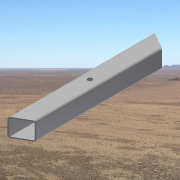
# Autodesk Inventor part: 2f2ao
Saved by Autodesk Inventor 2013 SP2 (Build 170200200, 200)
## iProperties
Company: HERA Project
Created: 2013-06-27
Part Number: 2f2ao
Material: Steel
Document SubType Name: Modeling
Designer: David DeBoer
Density: 7.85 g/cm^3
Mass: 221.444 g
Surface Area: 345.852 cm^2
Volume: 28.2094 cm^3
Description: Feed backplane support cross piece
Title: Backplane support piece
Author: David DeBoer
Autodesk Inventor part; units mm, degrees
ref_plane "YZ Plane" through (0, 0, 0) normal (1, 0, 0) x (0, 1, 0)
ref_plane "XZ Plane" through (0, 0, 0) normal (0, 1, 0) x (-1, 0, 0)
ref_plane "XY Plane" through (0, 0, 0) normal (0, 0, 1) x (1, 0, 0)
sketch "Sketch1" plane through (0, 0, 0) normal (0, 0, 1) x (1, 0, 0)
  line L0 (3.175, 0) -> (22.225, 0)
  line L1 (25.4, 3.175) -> (25.4, 22.225)
  line L2 (22.225, 25.4) -> (3.175, 25.4)
  line L3 (0, 22.225) -> (0, 3.175)
  arc A0 (3.175, 25.4) -> (0, 22.225) centre (3.175, 22.225) ccw
  arc A1 (0, 3.175) -> (3.175, 0) centre (3.175, 3.175) ccw
  arc A2 (22.225, 0) -> (25.4, 3.175) centre (22.225, 3.175) ccw
  arc A3 (25.4, 22.225) -> (22.225, 25.4) centre (22.225, 22.225) ccw
  line L4 (3.175, 23.749) -> (22.225, 23.749)
  arc A4 (23.749, 22.225) -> (22.225, 23.749) centre (22.225, 22.225) ccw
  line L5 (23.749, 22.225) -> (23.749, 3.175)
  arc A5 (22.225, 1.651) -> (23.749, 3.175) centre (22.225, 3.175) ccw
  line L6 (22.225, 1.651) -> (3.175, 1.651)
  arc A6 (1.651, 3.175) -> (3.175, 1.651) centre (3.175, 3.175) ccw
  line L7 (1.651, 3.175) -> (1.651, 22.225)
  arc A7 (3.175, 23.749) -> (1.651, 22.225) centre (3.175, 22.225) ccw
  point P0 (0, 0)
  point P1 (25.4, 0)
  point P2 (0, 25.4)
  dimension "d0" = 25.4
  dimension "d1" = 25.4
  dimension "d2" = 3.175
  dimension "d3" = 1.651
  constraints: 16 end point, 16 point on circle, 8 centre point, 8 tangent, 6 point on line, 4 parallel, 3 equal radius, 2 perpendicular, 1 horizontal, 7 other
  measures "d0" distance of point (0, 0) point (25.4, 0)
  measures "d1" distance of point (0, 25.4) point (0, 0)
  measures "d2" radius of A0
  measures "d3" distance between parallel lines of L4 L2
extrude "Extrusion1" add sketch "Sketch1" along normal blind 203.2
sketch "Sketch2" plane through (3.175, 25.4, 0) normal (0, 1, 0) x (1, 0, 0)
  line L0 (19.05, -203.2) -> (0, -203.2) projected
  line L1 (-3.175, 0) -> (22.2557, 0)
  line L2 (-3.175, 0) -> (32.385, 0) construction
  line L3 (22.2557, 0) -> (22.2557, -14.6824)
  line L4 (-3.175, 0) -> (22.2557, -14.6824)
  line L5 (-3.175, 0) -> (-3.175, -203.2) construction
  line L6 (-3.175, -101.6) -> (22.2557, -101.6) construction
  line L7 (-3.175, -203.2) -> (22.2557, -203.2)
  line L8 (22.2557, -203.2) -> (22.2557, -188.5176)
  line L9 (-3.175, -203.2) -> (22.2557, -188.5176)
  point P0 (0, 0)
  constraints: 18 end point, 2 parallel, 2 perpendicular, 2 symmetric about line, 1 horizontal, 1 midpoint
extrude "Extrusion2" cut sketch "Sketch2" against normal blind 203.2
sketch "Sketch3" plane through (3.175, 25.4, 201.3669) normal (0, 1, 0) x (1, 0, 0)
  line L0 (0, 199.5338) -> (0, 0) projected
  line L1 (19.05, 188.5353) -> (19.05, 10.9985) projected
  line L2 (0, 99.7669) -> (19.05, 99.7669) construction
  circle A0 centre (9.525, 99.7669) radius 2.5512
  point P0 (-3.175, 201.3669)
  constraints: 3 midpoint, 2 end point, 1 centre point
hole "Hole1" at (12.7, 25.4, 101.6) direction (0, -1, 0) diameter 6.35 end through all
body "Solid1"
